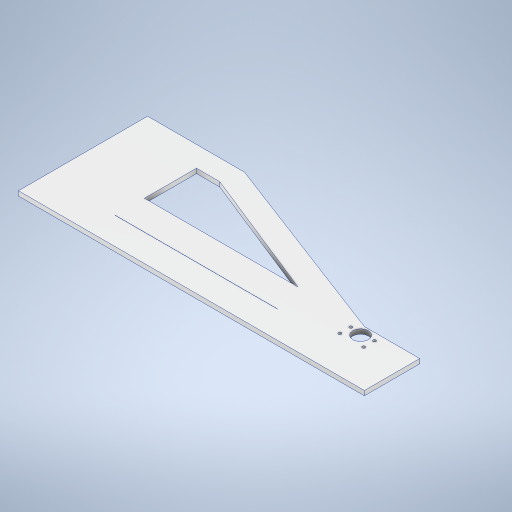
# Autodesk Inventor part: YFlanPlate
Saved by Autodesk Inventor 2024 (Build 280153000, 153)
## iProperties
Created: 2023-06-18
Part Number: YFlanPlate
Material: Aluminum 6061
Document SubType Name: Modeling
Designer: KirikDK
Mass: 3497.99 g
Surface Area: 2956.13 cm^2
Volume: 1295.55 cm^3
Density: 2.7 g/cm^3
Appearance: Aluminum - Flat
Author: KirikDK
Autodesk Inventor part; units mm, degrees
ref_plane "YZ Plane" through (0, 0, 0) normal (1, 0, 0) x (0, 1, 0)
ref_plane "XZ Plane" through (0, 0, 0) normal (0, 1, 0) x (-1, 0, 0)
ref_plane "XY Plane" through (0, 0, 0) normal (0, 0, 1) x (1, 0, 0)
sketch "Sketch3" plane through (0, 0, 0) normal (0, 1, 0) x (-1, 0, 0)
  line L0 (-219.2412, 70.0717) -> (200.7588, -89.9283)
  line L1 (205.7588, -63.9283) -> (-110.8967, 62.7339)
  line L2 (200.7588, -89.9283) -> (310.7588, -89.9283)
  line L3 (278.7588, -63.9283) -> (205.7588, -63.9283)
  line L4 (278.7588, 86.3746) -> (278.7588, -63.9283)
  line L5 (310.7588, -89.9283) -> (310.7588, 190.0717)
  line L6 (-110.8967, 86.3746) -> (278.7588, 86.3746)
  line L7 (278.7588, 112.3746) -> (-110.8967, 112.3746)
  line L8 (-110.8967, 150.1531) -> (278.7588, 150.1531)
  line L9 (278.7588, 150.1531) -> (278.7588, 112.3746)
  line L10 (-339.2412, 190.0717) -> (310.7588, 190.0717)
  line L11 (-110.8967, 112.3746) -> (-110.8967, 150.1531)
  line L12 (-339.2412, 70.0717) -> (-219.2412, 70.0717)
  line L13 (-339.2412, 70.0717) -> (-339.2412, 190.0717)
  circle A0 centre (-256.9912, 109.3217) radius 3.25
  circle A1 centre (-256.9912, 85.8217) radius 3.25
  circle A2 centre (-231.2412, 90.3217) radius 17
  circle A3 centre (-205.4912, 85.8217) radius 3.25
  circle A4 centre (-205.4912, 109.3217) radius 3.25
  line L14 (-110.8967, 86.3746) -> (-110.8967, 62.7339)
  line L15 (260, -45.1696) -> (209.3714, -45.1696)
  line L16 (209.3714, -45.1696) -> (-72.5921, 67.6158)
  line L17 (-72.5921, 67.6158) -> (260, 67.6158)
  line L18 (260, 67.6158) -> (260, -45.1696)
  line L19 (260, 131.1334) -> (-92.1379, 131.1334)
  line L20 (-92.1379, 131.1334) -> (-92.1379, 131.3943)
  line L21 (-92.1379, 131.3943) -> (260, 131.3943)
  line L22 (260, 131.3943) -> (260, 131.1334)
  point P0 (0, 0)
  constraints: 46 end point, 5 centre point, 1 vertical, 6 other
extrude "Extrusion2" add sketch "Sketch3" along normal blind 10 contours L12 L13 L10 L5 L2 L0 | L1 L14 L6 L4 L3 | L7 L11 L8 L9
sketch "Sketch4" plane through (-310.7588, 0, -89.9283) normal (-1, 0, 0) x (0, 0, 1)
  line L0 (0, 0) -> (280, 0) projected
  line L1 (280, 0) -> (280, 10) projected
  line L2 (0, 10) -> (280, 10) projected
  line L3 (0, 0) -> (0, 10) projected
  point P0 (89.9283, 0)
extrude "Extrusion3" add sketch "Sketch4" along normal blind 100
body "Solid2"
